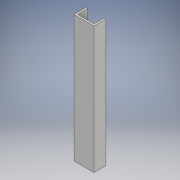
# Autodesk Inventor part: ceownik-pedal
Saved by Autodesk Inventor 2017 (Build 210142000, 142)
## iProperties
Created: 2017-03-23
Part Number: ceownik-pedal
Material: Aluminium
Document SubType Name: Modeling
Designer: Damian
Density: 2.7 g/cm^3
Appearance: Satynowy
Author: Damian
Autodesk Inventor part; units mm, degrees
ref_plane "YZ Plane" through (0, 0, 0) normal (1, 0, 0) x (0, 1, 0)
ref_plane "XZ Plane" through (0, 0, 0) normal (0, 1, 0) x (-1, 0, 0)
ref_plane "XY Plane" through (0, 0, 0) normal (0, 0, 1) x (1, 0, 0)
sketch "Szkic1" plane through (0, 0, 0) normal (0, 0, 1) x (1, 0, 0)
  line L0 (12.5, 0) -> (-12.5, 0)
  line L1 (-12.5, 0) -> (-12.5, 15)
  line L2 (12.5, 15) -> (12.5, 0)
  line L3 (-9.5, 2) -> (9.5, 2)
  line L4 (-12.5, 15) -> (-10.5, 15)
  line L5 (10.5, 15) -> (12.5, 15)
  line L6 (-10.5, 15) -> (-10.5, 3)
  line L7 (10.5, 3) -> (10.5, 15)
  arc A0 (-10.5, 3) -> (-9.5, 2) centre (-9.5, 3) ccw
  arc A1 (9.5, 2) -> (10.5, 3) centre (9.5, 3) ccw
  dimension "d2" = 25
  dimension "d3" = 15
  dimension "d5" = 1
  constraints: 16 end point, 4 parallel, 4 point on circle, 4 tangent, 2 centre point, 1 equal radius, 1 horizontal, 1 perpendicular, 1 vertical
  measures "d2" distance of L1.end L2.start
  measures "d3" distance of L0.end L1.end
  measures "d5" radius of A0
extrude "Wyciągnięcie proste1" add sketch "Szkic1" along normal mid plane 160
